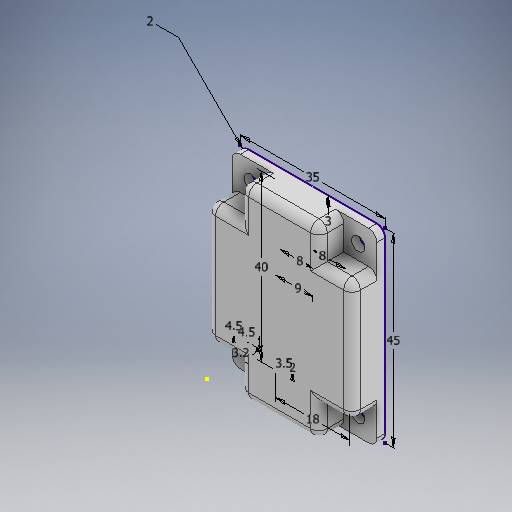
# Autodesk Inventor part: final sensor housing
Saved by Autodesk Inventor 2025.3 (Build 293356000, 356)
## iProperties
Created: 2026-04-08
Part Number: final sensor housing
Material: Generic
Document SubType Name: Modeling
Designer: user
Density: 1 g/cm^3
Appearance: Default
Author: user
## iProperties of the stored document final sensor housing_3DPrint.ipt
Created: 2026-04-12
Part Number: final sensor housing_3DPrint
Material: Generic
Document SubType Name: Modeling
Designer: user
Density: 1 g/cm^3
Appearance: Default
Author: user
Autodesk Inventor part; units mm, degrees
ref_plane "YZ Plane" through (0, 0, 0) normal (1, 0, 0) x (0, 1, 0)
ref_plane "XZ Plane" through (0, 0, 0) normal (0, 1, 0) x (-1, 0, 0)
ref_plane "XY Plane" through (0, 0, 0) normal (0, 0, 1) x (1, 0, 0)
sketch "Sketch1" plane through (0, 0, 0) normal (0, 0, 1) x (1, 0, 0)
  line L0 (2, 0) -> (33, 0)
  line L1 (35, 2) -> (35, 43)
  line L2 (33, 45) -> (2, 45)
  line L3 (0, 43) -> (0, 2)
  arc A0 (2, 45) -> (0, 43) centre (2, 43) ccw
  arc A1 (35, 43) -> (33, 45) centre (33, 43) ccw
  arc A2 (33, 0) -> (35, 2) centre (33, 2) ccw
  arc A3 (0, 2) -> (2, 0) centre (2, 2) ccw
  line L4 (17.5, 45) -> (17.5, 0) construction
  line L5 (26.5, 42) -> (8.5, 42)
  line L6 (8.5, 42) -> (8.5, 2)
  line L7 (8.5, 2) -> (26.5, 2)
  line L8 (26.5, 2) -> (26.5, 42)
  line L9 (9.5, 42) -> (25.5, 42)
  line L10 (25.5, 42) -> (25.5, 2)
  line L11 (25.5, 2) -> (9.5, 2)
  line L12 (9.5, 2) -> (9.5, 42)
  line L13 (8.5, 2) -> (12, 2)
  line L14 (12, 2) -> (12, 4)
  line L15 (12, 4) -> (8.5, 4)
  line L16 (8.5, 4) -> (8.5, 2)
  line L17 (23, 2) -> (23, 4)
  line L18 (23, 4) -> (26.5, 4)
  circle A4 centre (4.5, 4.5) radius 1.6
  circle A5 centre (30.5, 4.5) radius 1.6
  line L19 (35, 22.5) -> (0, 22.5)
  circle A6 centre (4.5, 40.5) radius 1.6
  circle A7 centre (30.5, 40.5) radius 1.6
  point P0 (0, 0)
  point P1 (35, 45)
  point P2 (35, 0)
  point P3 (0, 45)
  point P4 (17.5, 22.5)
  point P5 (25.5, 4)
  point P6 (9.5, 4)
  dimension "d0" = 35
  dimension "d1" = 45
  dimension "d2" = 2
  dimension "d5" = 18
  dimension "d6" = 40
  dimension "d7" = 9
  dimension "d8" = 3
  dimension "d9" = 8
  dimension "d10" = 8
  dimension "d11" = 3.5
  dimension "d12" = 2
  dimension "d31" = 3.2
  dimension "d35" = 4.5
  dimension "d36" = 4.5
  constraints: 40 end point, 10 point on line, 8 centre point, 8 parallel, 8 point on circle, 8 tangent, 6 symmetric about line, 5 midpoint, 4 horizontal, 4 perpendicular, 3 equal radius, 3 other
  measures "d0" distance of point (0, 45) point (35, 45)
  measures "d1" distance of point (35, 45) point (35, 0)
  measures "d2" radius of A0
  measures "d5" distance of L7.end L6.end
  measures "d6" distance of L6.end L5.end
  measures "d7" distance from line of point (17.5, 22.5) L6
  measures "d8" distance between parallel lines of L5 L2
  measures "d9" distance between parallel lines of L4 L12
  measures "d10" distance between parallel lines of L4 L10
  measures "d11" distance of L14.end L15.end
  measures "d12" distance of L13.end L14.end
  measures "d31" diameter of A4
  measures "d35" distance from line of L3 A4.centre
  measures "d36" distance from line of L0 A4.centre
extrude "Extrusion1" add sketch "Sketch1" along normal blind 8 contours A3 L3 L19 L6 L7 L8 L1 A2 L0 | L3 A0 L2 A1 L1 L19 L8 L5 L6 | L19 L12 L15 L6 | L6 L5 L12 L19 | L19 L10 L5 L8 | L8 L18 L10 L19 | L15 L12 L7 L6 | L19 L10 L18 L17 L7 L14 L15 L12 | L12 L5 L10 L19 | L8 L7 L10 L18 | L15 L14 L7 L12 | L10 L7 L17 L18 | A4 | A5 | A6 | A7
sketch "Sketch2" plane through (0, 0, 8) normal (0, 0, 1) x (1, 0, 0)
  point P0 (0, 0)
extrude "Extrusion2" cut sketch "Sketch1" along normal blind 6 contours L19 L10 L18 L17 L7 L14 L15 L12 | L12 L5 L10 L19
sketch "Sketch3" plane through (0, 0, 8) normal (0, 0, 1) x (1, 0, 0)
  line L0 (35, 0) -> (27, 0)
  line L1 (27, 0) -> (27, 8)
  line L2 (27, 8) -> (35, 8)
  line L3 (35, 8) -> (35, 0)
  line L4 (0, 43) -> (0, 2) projected
  line L5 (2, 0) -> (33, 0) projected
  line L6 (17.5, 0) -> (17.5, 45)
  line L7 (33, 45) -> (2, 45) projected
  line L8 (0, 22.5) -> (35, 22.5)
  line L9 (0, 0) -> (8, 0)
  line L10 (8, 0) -> (8, 8)
  line L11 (8, 8) -> (0, 8)
  line L12 (0, 8) -> (0, 0)
  line L13 (33, 0) -> (2, 0)
  line L14 (35, 45) -> (27, 45)
  line L15 (27, 45) -> (27, 37)
  line L16 (27, 37) -> (35, 37)
  line L17 (35, 37) -> (35, 45)
  line L18 (2, 45) -> (33, 45)
  line L19 (0, 45) -> (8, 45)
  line L20 (8, 45) -> (8, 37)
  line L21 (8, 37) -> (0, 37)
  line L22 (0, 37) -> (0, 45)
  line L23 (33, 45) -> (2, 45)
  point P0 (0, 2)
  dimension "d37" = 8
  dimension "d38" = 8
  dimension "d39" = 35
  constraints: 42 end point, 18 symmetric about line, 3 midpoint, 2 horizontal, 2 parallel, 1 perpendicular
  measures "d37" distance of L1.end L2.end
  measures "d38" distance of L0.end L1.end
  measures "d39" distance from line of L0.start L4
extrude "Extrusion3" cut sketch "Sketch3" against normal blind 6 contours L0 L1 L2 L3 | L22 L19 L7 L20 L21 L4 | L11 L10 L5 L9 L12 L4 | L14 L17 L16 L15 L7
extrude "Extrusion4" cut sketch "Sketch1" along normal blind 6 contours A4 | A5 | A6 | A7
fillet "Fillet1" radius 2 4 edges at (17.5, 45, 8) (35, 22.5, 8) (0, 22.5, 8) (17.5, 0, 8)
sketch "Sketch4" plane through (12, 2, 0) normal (0, 1, 0) x (1, 0, 0)
  line L0 (-10, 0) -> (21, 0) projected
  line L1 (11, -6) -> (0, -6)
  line L2 (0, -6) -> (0, 0)
  line L3 (0, 0) -> (11, 0)
  line L4 (11, 0) -> (11, -6)
  point P0 (-12, 0)
  constraints: 8 end point, 2 parallel, 1 horizontal, 1 perpendicular, 1 point on line
extrude "Extrusion5" cut sketch "Sketch4" against normal through all
fillet "Fillet2" radius 2 6 edges at (27, 44.4142, 7.4142) (27, 45, 4) (27, 40, 8) (34.4142, 37, 7.4142) (35, 37, 4) (30, 37, 8)
fillet "Fillet3" radius 2 18 edges at (8, 44.4142, 7.4142) (8, 45, 4) (8, 40, 8) (0.5858, 37, 7.4142) (0, 37, 4) (5, 37, 8) (0.5858, 8, 7.4142) (0, 8, 4) (5, 8, 8) (8, 0.5858, 7.4142) (8, 0, 4) (8, 5, 8) (34.4142, 8, 7.4142) (35, 8, 4) (30, 8, 8) (27, 0.5858, 7.4142) (27, 0, 4) (27, 5, 8)
body "Solid1"
